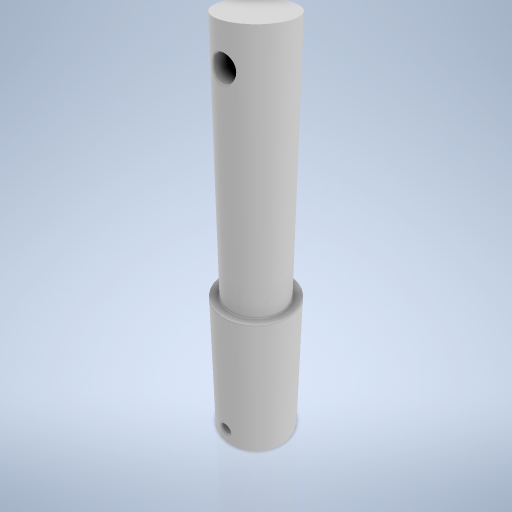
# Autodesk Inventor part: 18
Saved by Autodesk Inventor 2024.2 (Build 282272000, 272)
## iProperties
Created: 2024-05-05
Part Number: 18
Material: Generisch
Document SubType Name: Modeling
Designer: Fabri
Density: 1 g/cm^3
Appearance: Vorgabe
Author: Fabri
Autodesk Inventor part; units mm, degrees
ref_plane "YZ Plane" through (0, 0, 0) normal (1, 0, 0) x (0, 1, 0)
ref_plane "XY Plane" through (0, 0, 0) normal (0, 0, 1) x (1, 0, 0)
sketch "Skizze1" plane through (0, 0, 0) normal (0, 1, 0) x (-1, 0, 0)
  line L0 (0, 0) -> (14, 0)
  line L1 (14, 0) -> (14, -23)
  line L2 (14, -23) -> (14, -23)
  line L3 (14, -23) -> (14, -33)
  line L4 (14, -33) -> (14, -33)
  line L5 (14, -33) -> (14, -106)
  line L6 (14, -106) -> (18, -106)
  line L7 (18, -106) -> (18, -165)
  line L8 (18, -165) -> (18, -165)
  line L9 (18, -165) -> (18, -171)
  line L10 (18, -171) -> (18, -171)
  line L11 (18, -171) -> (18, -176)
  line L12 (18, -176) -> (0, -176)
  line L13 (0, -176) -> (0, 0)
  point P0 (18, -168)
  point P1 (18, -173.5)
  point P2 (14, -28)
  dimension "d3" = 36
  dimension "d6" = 78
  dimension "d8" = 28
  dimension "d12" = 176
  dimension "d13" = 36
  dimension "d14" = 70
  constraints: 28 end point, 11 perpendicular, 4 point on line, 3 midpoint, 1 coincident, 1 horizontal, 1 vertical alignment
  measures "d3" diameter of point (18, -173.5) L13
  measures "d6" distance from line of L6 point (14, -28)
  measures "d8" diameter of L1 L13
  measures "d12" distance between parallel lines of L12 L0
  measures "d13" diameter of L7 L13
  measures "d14" distance between parallel lines of L12 L6
revolve "Umdrehung1" add sketch "Skizze1" angle 360 about axis through (0, 0, -176) along (0, 0, 1)
ref_plane "Arbeitsebene1" through (0, 18, 0) normal (0, 1, 0) x (-1, 0, 0)
sketch "Skizze2" plane through (0, 18, 0) normal (0, 1, 0) x (-1, 0, 0)
  line L0 (18, -106) -> (-18, -106) projected
  line L1 (18, -176) -> (-18, -176) projected
  line L2 (14, 0) -> (-14, 0) projected
  point P0 (0, 0)
  point P1 (0, -168)
  point P2 (0, -176)
  point P3 (0, -14)
  dimension "d16" = 8
  dimension "d17" = 14
  constraints: 2 vertical alignment, 1 midpoint
  measures "d16" distance of point (0, -168) point (0, -176)
  measures "d17" distance of point (0, 0) point (0, -14)
hole "Bohrung1" at (0, 18, -168) direction (0, -1, 0) diameter 6 end through all
hole "Bohrung2" at (0, 18, -14) direction (0, -1, 0) diameter 10 end through all
